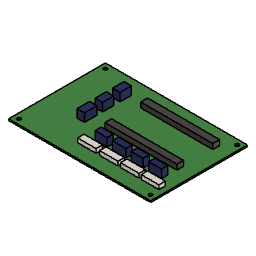
pcb v3 (Autodesk Fusion 360 design; units mm, degrees)
Autodesk Fusion 360 part; units mm, degrees
sketch "草图1" plane through (0, 0, 0) normal (0, 0, 1) x (1, 0, 0)
  line L0 (0, 0) -> (138, 0)
  line L1 (138, 0) -> (138, 94)
  line L2 (138, 94) -> (0, 94)
  line L3 (0, 94) -> (0, 0)
  line L4 (-20, 47) -> (170, 47)
  line L5 (69, 129.1488) -> (69, -36.2993)
  circle A0 centre (5, 89) radius 1.75
  circle A1 centre (133, 89) radius 1.75
  circle A2 centre (5, 5) radius 1.75
  circle A3 centre (133, 5) radius 1.75
  dimension "d1" = 94
  dimension "d2" = 138
  dimension "d3" = 84
  dimension "d4" = 128
  dimension "d5" = 3.5
  constraint horizontal L0
  constraint vertical L1
  constraint horizontal L2
  constraint vertical L3
  constraint coincident L0.start L3.end
  constraint perpendicular L1 L4
  constraint perpendicular L4 L5
  constraint symmetric L0 L2 L4
  constraint symmetric L5 A0 A1
  constraint symmetric L4 A0 A2
  constraint symmetric L4 A1 A3
  measures "d1" distance of L0.start L2.end
  measures "d2" distance of L1.end L2.end
  measures "d3" distance of A0.centre A2.centre
  measures "d4" distance of A0.centre A1.centre
  measures "d5" diameter of A0
extrude "拉伸1" add sketch "草图1" along normal blind 1.5 makes body 1
sketch "草图2" plane through (0, 0, 1.5) normal (0, 0, 1) x (-1, 0, 0)
  circle A0 centre (-5, -5) radius 1.75
  circle A1 centre (-133, -89) radius 1.75
  circle A2 centre (-133, -5) radius 1.75
  circle A3 centre (-5, -89) radius 1.75
  line L0 (0, -94) -> (0, 0)
  line L1 (0, 0) -> (-138, 0)
  line L2 (-138, 0) -> (-138, -94)
  line L3 (-138, -94) -> (0, -94)
  line L4 (-55, -80) -> (-125.0378, -80)
  line L5 (-125.0378, -80) -> (-125.0378, -73.349)
  line L6 (-125.0378, -73.349) -> (-55, -73.349)
  line L7 (-55, -73.349) -> (-55, -80)
  line L8 (-55, -45) -> (-125.0378, -45)
  line L9 (-125.0378, -45) -> (-125.0378, -38.5504)
  line L10 (-125.0378, -38.5504) -> (-55, -38.5504)
  line L11 (-55, -38.5504) -> (-55, -45)
  constraint horizontal L4
  constraint vertical L5
  constraint horizontal L6
  constraint vertical L7
  constraint horizontal L8
  constraint vertical L9
  constraint horizontal L10
  constraint vertical L11
extrude "拉伸2" add sketch "草图2" along normal blind 5 separate body contours L4 L5 L6 L7 | L8 L9 L10 L11 makes body 2 at (101.6919, 75.566, 1.5) makes body 3 at (78.3459, 42.8501, 1.5)
sketch "草图3" plane through (0, 0, 1.5) normal (0, 0, 1) x (-1, 0, 0)
  circle A0 centre (-5, -5) radius 1.75
  circle A1 centre (-133, -89) radius 1.75
  circle A2 centre (-133, -5) radius 1.75
  circle A3 centre (-5, -89) radius 1.75
  line L0 (0, -94) -> (0, 0)
  line L1 (0, 0) -> (-138, 0)
  line L2 (-138, 0) -> (-138, -94)
  line L3 (-138, -94) -> (0, -94)
  line L4 (-60, -30) -> (-71.7172, -30)
  line L5 (-71.7172, -30) -> (-71.7172, -24.0385)
  line L6 (-71.7172, -24.0385) -> (-60, -24.0385)
  line L7 (-60, -24.0385) -> (-60, -30)
  line L8 (-76.8041, -30) -> (-90.0303, -30)
  line L9 (-90.0303, -30) -> (-90.0303, -24.0385)
  line L10 (-90.0303, -24.0385) -> (-76.8041, -24.0385)
  line L11 (-76.8041, -24.0385) -> (-76.8041, -30)
  line L12 (-95, -30) -> (-106.7446, -30)
  line L13 (-106.7446, -30) -> (-106.7446, -24.0385)
  line L14 (-106.7446, -24.0385) -> (-95, -24.0385)
  line L15 (-95, -24.0385) -> (-95, -30)
  line L16 (-112.1223, -30) -> (-124.6217, -30)
  line L17 (-124.6217, -30) -> (-124.6217, -24.0385)
  line L18 (-124.6217, -24.0385) -> (-112.1223, -24.0385)
  line L19 (-112.1223, -24.0385) -> (-112.1223, -30)
  constraint horizontal L4
  constraint vertical L5
  constraint horizontal L6
  constraint vertical L7
  constraint horizontal L8
  constraint vertical L9
  constraint horizontal L10
  constraint vertical L11
  constraint horizontal L12
  constraint vertical L13
  constraint horizontal L14
  constraint vertical L15
  constraint horizontal L16
  constraint vertical L17
  constraint horizontal L18
  constraint vertical L19
extrude "拉伸3" add sketch "草图3" along normal blind 8 separate body contours L4 L5 L6 L7 | L8 L9 L10 L11 | L12 L13 L14 L15 | L16 L17 L18 L19 makes body 4 at (98.9149, 30, 4.1667) makes body 5 at (81.2129, 30, 4.1667) makes body 6 at (116.2887, 30, 6.8333) makes body 7 at (63.9057, 30, 4.1667)
sketch "草图4" plane through (0, 0, 1.5) normal (0, 0, 1) x (-1, 0, 0)
  circle A0 centre (-5, -5) radius 1.75
  circle A1 centre (-133, -89) radius 1.75
  circle A2 centre (-133, -5) radius 1.75
  circle A3 centre (-5, -89) radius 1.75
  line L0 (0, -94) -> (0, 0)
  line L1 (0, 0) -> (-138, 0)
  line L2 (-138, 0) -> (-138, -94)
  line L3 (-138, -94) -> (0, -94)
  line L4 (-53.6424, -19.7138) -> (-71.5683, -19.7138)
  line L5 (-71.5683, -19.7138) -> (-71.5683, -13.4321)
  line L6 (-71.5683, -13.4321) -> (-53.6424, -13.4321)
  line L7 (-53.6424, -13.4321) -> (-53.6424, -19.7138)
  line L8 (-74.9389, -19.7138) -> (-92.8648, -19.7138)
  line L9 (-92.8648, -19.7138) -> (-92.8648, -13.4321)
  line L10 (-92.8648, -13.4321) -> (-74.9389, -13.4321)
  line L11 (-74.9389, -13.4321) -> (-74.9389, -19.7138)
  line L12 (-95.3162, -19.7138) -> (-113.2421, -19.7138)
  line L13 (-113.2421, -19.7138) -> (-113.2421, -13.4321)
  line L14 (-113.2421, -13.4321) -> (-95.3162, -13.4321)
  line L15 (-95.3162, -13.4321) -> (-95.3162, -19.7138)
  line L16 (-115.387, -19.7138) -> (-132.5468, -19.7138)
  line L17 (-132.5468, -19.7138) -> (-132.5468, -13.4321)
  line L18 (-132.5468, -13.4321) -> (-115.387, -13.4321)
  line L19 (-115.387, -13.4321) -> (-115.387, -19.7138)
  constraint horizontal L4
  constraint vertical L5
  constraint horizontal L6
  constraint vertical L7
  constraint horizontal L8
  constraint vertical L9
  constraint horizontal L10
  constraint vertical L11
  constraint horizontal L12
  constraint vertical L13
  constraint horizontal L14
  constraint vertical L15
  constraint horizontal L16
  constraint vertical L17
  constraint horizontal L18
  constraint vertical L19
extrude "拉伸4" add sketch "草图4" along normal blind 4 separate body contours L4 L5 L6 L7 | L8 L9 L10 L11 | L12 L13 L14 L15 | L16 L17 L18 L19 makes body 8 at (101.2915, 15.526, 1.5) makes body 9 at (86.8895, 17.6199, 1.5) makes body 10 at (121.107, 15.526, 1.5) makes body 11 at (59.6177, 15.526, 1.5)
sketch "草图5" plane through (0, 0, 1.5) normal (0, 0, 1) x (-1, 0, 0)
  circle A0 centre (-5, -5) radius 1.75
  circle A1 centre (-133, -89) radius 1.75
  circle A2 centre (-133, -5) radius 1.75
  circle A3 centre (-5, -89) radius 1.75
  line L0 (0, -94) -> (0, 0)
  line L1 (0, 0) -> (-138, 0)
  line L2 (-138, 0) -> (-138, -94)
  line L3 (-138, -94) -> (0, -94)
  line L4 (-32.6944, -79.3897) -> (-39.8832, -79.3897)
  line L5 (-39.8832, -79.3897) -> (-39.8832, -68.3771)
  line L6 (-39.8832, -68.3771) -> (-32.6944, -68.3771)
  line L7 (-32.6944, -68.3771) -> (-32.6944, -79.3897)
  line L8 (-32.6944, -62.2589) -> (-39.8832, -62.2589)
  line L9 (-39.8832, -62.2589) -> (-39.8832, -51.3992)
  line L10 (-39.8832, -51.3992) -> (-32.6944, -51.3992)
  line L11 (-32.6944, -51.3992) -> (-32.6944, -62.2589)
  line L12 (-32.6944, -46.0458) -> (-39.8832, -46.0458)
  line L13 (-39.8832, -46.0458) -> (-39.8832, -33.8095)
  line L14 (-39.8832, -33.8095) -> (-32.6944, -33.8095)
  line L15 (-32.6944, -33.8095) -> (-32.6944, -46.0458)
  constraint horizontal L4
  constraint vertical L5
  constraint horizontal L6
  constraint vertical L7
  constraint horizontal L8
  constraint vertical L9
  constraint horizontal L10
  constraint vertical L11
  constraint horizontal L12
  constraint vertical L13
  constraint horizontal L14
  constraint vertical L15
extrude "拉伸5" add sketch "草图5" along normal blind 8 separate body contours L4 L5 L6 L7 | L8 L9 L10 L11 | L12 L13 L14 L15 makes body 12 at (32.6944, 37.8883, 6.8333) makes body 13 at (39.8832, 58.639, 4.1667) makes body 14 at (39.8832, 75.7189, 4.1667)
copy_body "实体->零部件1" bodies 1 removing the originals makes body 15 in component "Component"
copy_body "实体->零部件2" bodies 2 removing the originals makes body 16 in component "Component'"
copy_body "实体->零部件3" bodies 3 removing the originals makes body 17 in component "Component''"
copy_body "实体->零部件4" bodies 4 removing the originals makes body 18 in component "Component'''"
copy_body "实体->零部件5" bodies 5 removing the originals makes body 19 in component "Component''''"
copy_body "实体->零部件6" bodies 6 removing the originals makes body 20 in component "Component'''''"
copy_body "实体->零部件7" bodies 7 removing the originals makes body 21 in component "Component''''''"
copy_body "实体->零部件8" bodies 8 removing the originals makes body 22 in component "Component'''''''"
copy_body "实体->零部件9" bodies 9 removing the originals makes body 23 in component "Component''''''''"
copy_body "实体->零部件10" bodies 10 removing the originals makes body 24 in component "Component'''''''''"
copy_body "实体->零部件11" bodies 11 removing the originals makes body 25 in component "Component''''''''''"
copy_body "实体->零部件12" bodies 12 removing the originals makes body 26 in component "Component'''''''''''"
copy_body "实体->零部件13" bodies 13 removing the originals makes body 27 in component "Component''''''''''''"
copy_body "实体->零部件14" bodies 14 removing the originals makes body 28 in component "Component'''''''''''''"
component "Component" placed x (1, 0, 0) y (0, 1, 0) z (0, 0, 1) at (0, 0, 0)
component "Component'" placed x (1, 0, 0) y (0, 1, 0) z (0, 0, 1) at (0, 0, 0)
component "Component''" placed x (1, 0, 0) y (0, 1, 0) z (0, 0, 1) at (0, 0, 0)
component "Component'''" placed x (1, 0, 0) y (0, 1, 0) z (0, 0, 1) at (0, 0, 0)
component "Component''''" placed x (1, 0, 0) y (0, 1, 0) z (0, 0, 1) at (0, 0, 0)
component "Component'''''" placed x (1, 0, 0) y (0, 1, 0) z (0, 0, 1) at (0, 0, 0)
component "Component''''''" placed x (1, 0, 0) y (0, 1, 0) z (0, 0, 1) at (0, 0, 0)
component "Component'''''''" placed x (1, 0, 0) y (0, 1, 0) z (0, 0, 1) at (0, 0, 0)
component "Component''''''''" placed x (1, 0, 0) y (0, 1, 0) z (0, 0, 1) at (0, 0, 0)
component "Component'''''''''" placed x (1, 0, 0) y (0, 1, 0) z (0, 0, 1) at (0, 0, 0)
component "Component''''''''''" placed x (1, 0, 0) y (0, 1, 0) z (0, 0, 1) at (0, 0, 0)
component "Component'''''''''''" placed x (1, 0, 0) y (0, 1, 0) z (0, 0, 1) at (0, 0, 0)
component "Component''''''''''''" placed x (1, 0, 0) y (0, 1, 0) z (0, 0, 1) at (0, 0, 0)
component "Component'''''''''''''" placed x (1, 0, 0) y (0, 1, 0) z (0, 0, 1) at (0, 0, 0)
